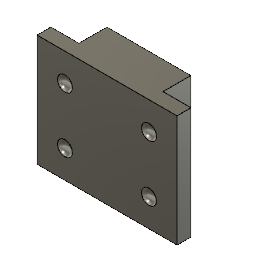
Open-JIP Plant Back Panel v1 (Autodesk Fusion 360 design; units mm, degrees)
Autodesk Fusion 360 part; units mm, degrees
sketch "Sketch1" plane through (0, 0, 0) normal (0, 1, 0) x (1, 0, 0)
  line L0 (0, 0) -> (100, 0)
  line L1 (100, 0) -> (100, 40)
  line L2 (100, 40) -> (0, 40)
  line L3 (0, 40) -> (0, 0)
  dimension "d1" = 100
  dimension "d2" = 40
  constraint horizontal L0
  constraint vertical L1
  constraint horizontal L2
  constraint vertical L3
  constraint coincident L0.start L3.end
  measures "d1" distance of L1.end L2.end
  measures "d2" distance of L0.end L1.end
extrude "Extrude1" add sketch "Sketch1" along normal blind 5 makes body 1
sketch "Sketch2" plane through (0, 5, 0) normal (0, 1, 0) x (-1, 0, 0)
  line L0 (0, -40) -> (0, 0)
  line L1 (0, 0) -> (-100, 0)
  line L2 (-100, 0) -> (-100, -40)
  line L3 (-100, -40) -> (0, -40)
  line L4 (0, -40) -> (-10, -40)
  line L5 (-10, -40) -> (-10, 0)
  line L6 (-10, 0) -> (0, 0)
  line L7 (0, 0) -> (0, -40)
  dimension "d5" = 10
  constraint horizontal L4
  constraint vertical L5
  constraint horizontal L6
  constraint vertical L7
  constraint coincident L1 L5.end
  constraint coincident L0.start L3.end
  measures "d5" distance of L0.start L4.end
extrude "Extrude2" add sketch "Sketch2" along normal blind 3 contours L0 L1 L3 L4 L5 L6 L7 bodies 1
sketch "Sketch3" plane through (0, 8, 0) normal (0, 1, 0) x (-1, 0, 0)
  line L0 (0, 0) -> (-10, 0)
  line L1 (-10, 0) -> (-10, -40)
  line L2 (-10, -40) -> (0, -40)
  line L3 (0, -40) -> (0, 0)
  line L4 (0, -40) -> (-100, -40)
  line L5 (-100, -40) -> (-100, 0)
  line L6 (-100, 0) -> (0, 0)
  line L7 (0, 0) -> (0, -40)
  point P0 (-100, 0)
  constraint horizontal L4
  constraint vertical L5
  constraint horizontal L6
  constraint vertical L7
  constraint coincident P0 L5.end
  constraint coincident L2.end L3.start
extrude "Extrude3" add sketch "Sketch3" along normal blind 6 bodies 1
sketch "Sketch4" plane through (100, 0, 0) normal (1, 0, 0) x (0, 0, -1)
  line L0 (0, 8) -> (40, 8)
  line L1 (40, 8) -> (40, 14)
  line L2 (40, 14) -> (0, 14)
  line L3 (0, 14) -> (0, 8)
  line L4 (2, 13) -> (38, 13)
  line L5 (38, 13) -> (38, 9)
  line L6 (38, 9) -> (2, 9)
  line L7 (2, 9) -> (2, 13)
  dimension "d10" = 4
  dimension "d11" = 2
  dimension "d12" = 2
  dimension "d13" = 1
  constraint horizontal L4
  constraint vertical L5
  constraint horizontal L6
  constraint vertical L7
  measures "d10" distance of L4.start L6.end
  measures "d11" distance of L1 L5
  measures "d12" distance of L3 L7
  measures "d13" distance of L0 L6
extrude "Extrude4" cut sketch "Sketch4" against normal blind 90 contours L4 L5 L6 L7 bodies 1
sketch "Sketch5" plane through (0, 14, 0) normal (0, 1, 0) x (-1, 0, 0)
  line L0 (0, 0) -> (-100, 0)
  line L1 (-100, 0) -> (-100, -40)
  line L2 (-100, -40) -> (0, -40)
  line L3 (0, -40) -> (0, 0)
  circle A0 centre (-55, -20) radius 7.5
  dimension "d16" = 20
  dimension "d17" = 15
  dimension "d18" = 55
  measures "d16" distance of L2 A0.centre
  measures "d17" diameter of A0
  measures "d18" distance of L3 A0.centre
extrude "Extrude5" cut sketch "Sketch5" against normal blind 8 contours A0 bodies 1
sketch "Sketch6" plane through (0, 14, 0) normal (0, 1, 0) x (-1, 0, 0)
  circle A0 centre (-55, -20) radius 7.5
  line L0 (0, 0) -> (-100, 0)
  line L1 (-100, 0) -> (-100, -40)
  line L2 (-100, -40) -> (0, -40)
  line L3 (0, -40) -> (0, 0)
  circle A1 centre (-55, -20) radius 15
  dimension "d21" = 30
  constraint concentric A0 A1
  measures "d21" diameter of A1
extrude "Extrude6" cut sketch "Sketch6" against normal blind 2 contours A1 bodies 1
extrude "Extrude7" add 1 faces at (10, 11.6667, -14) along direction (1, 0, 0) blind 90 on bodies 1 bodies 1
sketch "Sketch7" plane through (0, 0, -40) normal (0, 0, -1) x (-1, 0, 0)
  line L0 (-100, 0) -> (0, 0)
  line L1 (0, 0) -> (0, 14)
  line L2 (0, 14) -> (-100, 14)
  line L3 (-100, 14) -> (-100, 8)
  line L4 (-100, 8) -> (-10, 8)
  line L5 (-10, 8) -> (-10, 5)
  line L6 (-10, 5) -> (-100, 5)
  line L7 (-100, 5) -> (-100, 0)
  line L8 (-80, 12.5) -> (-30, 12.5)
  line L9 (-30, 12.5) -> (-30, 9.5)
  line L10 (-30, 9.5) -> (-80, 9.5)
  line L11 (-80, 9.5) -> (-80, 12.5)
  dimension "d26" = 1.5
  dimension "d27" = 1.5
  dimension "d28" = 20
  dimension "d29" = 30
  constraint horizontal L8
  constraint vertical L9
  constraint horizontal L10
  constraint vertical L11
  measures "d26" distance of L4 L10
  measures "d27" distance of L2 L8
  measures "d28" distance of L3 L11
  measures "d29" distance of L1 L9
extrude "Extrude8" cut sketch "Sketch7" against normal blind 37 contours L8 L9 L10 L11 bodies 1
extrude "Extrude9" cut 1 faces at (55.8396, 13, -15.821) along direction (0, -1, 0) blind 1 on bodies 1 bodies 1
sketch "Sketch8" plane through (0, 9.5, 0) normal (0, 1, 0) x (-1, 0, 0)
  line L0 (-80, -40) -> (-30, -40)
  line L1 (-30, -40) -> (-30, -3)
  line L2 (-30, -3) -> (-80, -3)
  line L3 (-80, -3) -> (-80, -40)
  circle A0 centre (-55, -20) radius 7.5
extrude "Extrude10" cut sketch "Sketch8" against normal blind 2 contours A0 bodies 1
move_body "Move1" bodies 1 to x (1, 0, 0) y (0, 0, 1) z (0, -1, 0) at (0, 0, -40)
move_body "Move2" bodies 1 to x (1, 0, 0) y (0, 1, 0) z (0, 0, 1) at (0, 0, 25)
sketch "Sketch9" plane through (0, 0, -15) normal (0, 0, -1) x (-1, 0, 0)
  line L0 (0, 0) -> (0, 40)
  line L1 (0, 40) -> (-100, 40)
  line L2 (-100, 40) -> (-100, 0)
  line L3 (-100, 0) -> (0, 0)
  circle A0 centre (-70, 30) radius 2.5
  circle A1 centre (-40, 30) radius 2.5
  circle A2 centre (-40, 10) radius 2.5
  circle A3 centre (-70, 10) radius 2.5
  dimension "d36" = 5
  dimension "d37" = 5
  dimension "d38" = 5
  dimension "d39" = 5
  dimension "d40" = 20
  dimension "d41" = 20
  dimension "d42" = 30
  dimension "d43" = 30
  dimension "d44" = 10
  dimension "d45" = 30
  measures "d36" diameter of A3
  measures "d37" diameter of A0
  measures "d38" diameter of A1
  measures "d39" diameter of A2
  measures "d40" distance of A1.centre A2.centre
  measures "d41" distance of A0.centre A3.centre
  measures "d42" distance of A0.centre A1.centre
  measures "d43" distance of A2.centre A3.centre
  measures "d44" distance of L3 A3.centre
  measures "d45" distance of L2 A3.centre
extrude "Extrude11" add sketch "Sketch9" along normal blind 2 contours A0 | A1 | A2 | A3 bodies 1
sketch "Sketch1 (2)" plane through (0, 0, 0) normal (0, 1, 0) x (1, 0, 0) in component "Attachment for IRWIN QuickGrip v0 v1"
  line L0 (0, 0) -> (40, 0)
  line L1 (40, 0) -> (40, 30)
  line L2 (40, 30) -> (0, 30)
  line L3 (0, 30) -> (0, 0)
  constraint horizontal L0
  constraint vertical L1
  constraint horizontal L2
  constraint vertical L3
  constraint coincident L0.start L3.end
extrude "Extrude1'" add sketch "Sketch1 (2)" along normal blind 10 separate body makes body 2 in component "Attachment for IRWIN QuickGrip v0 v1"
sketch "Sketch2 (2)" plane through (40, 0, 0) normal (1, 0, 0) x (0, 0, -1) in component "Attachment for IRWIN QuickGrip v0 v1"
  line L0 (0, 0) -> (30, 0)
  line L1 (30, 0) -> (30, 10)
  line L2 (30, 10) -> (0, 10)
  line L3 (0, 10) -> (0, 0)
  line L4 (7.3, 10) -> (22.7, 10)
  line L5 (22.7, 10) -> (22.7, 5.5)
  line L6 (22.7, 5.5) -> (7.3, 5.5)
  line L7 (7.3, 5.5) -> (7.3, 10)
  dimension "d3_1" = 15.4
  dimension "d4_1" = 4.5
  dimension "d5_1" = 7.3
  constraint horizontal L4
  constraint vertical L5
  constraint horizontal L6
  constraint vertical L7
  constraint collinear L2 L4
  measures "d3_1" distance of L5.end L6.end
  measures "d4_1" distance of L4.end L5.end
  measures "d5_1" distance of L3 L7
extrude "Extrude2'" cut sketch "Sketch2 (2)" against normal blind 35 contours L2 L4 L5 L6 L7 bodies 2 in component "Attachment for IRWIN QuickGrip v0 v1"
sketch "Sketch3 (2)" plane through (40, 0, 0) normal (1, 0, 0) x (0, 0, -1) in component "Attachment for IRWIN QuickGrip v0 v1"
  line L0 (7.3, 5.5) -> (7.3, 10)
  line L1 (7.3, 10) -> (0, 10)
  line L2 (0, 10) -> (0, 0)
  line L3 (0, 0) -> (30, 0)
  line L4 (30, 0) -> (30, 10)
  line L5 (30, 10) -> (22.7, 10)
  line L6 (22.7, 10) -> (22.7, 5.5)
  line L7 (22.7, 5.5) -> (7.3, 5.5)
  line L8 (4.5, 5.5) -> (25.5, 5.5)
  line L9 (25.5, 5.5) -> (25.5, 1.2)
  line L10 (25.5, 1.2) -> (4.5, 1.2)
  line L11 (4.5, 1.2) -> (4.5, 5.5)
  dimension "d8_1" = 21
  dimension "d9_1" = 4.5
  dimension "d10_1" = 4.3
  constraint horizontal L8
  constraint vertical L9
  constraint horizontal L10
  constraint vertical L11
  constraint collinear L7 L8
  measures "d8_1" distance of L9 L11
  measures "d9_1" distance of L2 L11
  measures "d10_1" distance of L8.end L9.end
extrude "Extrude3'" cut sketch "Sketch3 (2)" against normal blind 38 contours L7 L8 L9 L10 L11 bodies 2 in component "Attachment for IRWIN QuickGrip v0 v1"
sketch "Sketch10" plane through (0, 0, -76.0627) normal (0, 0, 1) x (1, 0, 0)
  line L0 (68.8222, 42.7595) -> (38.8222, 42.7595)
  line L1 (38.8222, 42.7595) -> (38.8222, 2.7595)
  line L2 (38.8222, 2.7595) -> (68.8222, 2.7595)
  line L3 (68.8222, 2.7595) -> (68.8222, 42.7595)
  line L4 (28.8222, 42.7595) -> (78.8222, 42.7595)
  line L5 (78.8222, 42.7595) -> (78.8222, 2.7595)
  line L6 (78.8222, 2.7595) -> (28.8222, 2.7595)
  line L7 (28.8222, 2.7595) -> (28.8222, 42.7595)
  dimension "d48" = 40
  dimension "d49" = 10
  dimension "d50" = 10
  constraint horizontal L4
  constraint vertical L5
  constraint horizontal L6
  constraint vertical L7
  measures "d48" distance of L4.end L5.end
  measures "d49" distance of L3 L5
  measures "d50" distance of L1 L7
extrude "Extrude4'" add sketch "Sketch10" along normal blind 5 sketch seen with x (0, 0, 1) y (-1, 0, 0) z (0, -1, 0) at (42.7595, -76.0627, -68.8222) bodies 2 in component "Attachment for IRWIN QuickGrip v0 v1"
sketch "Sketch11" plane through (0, 0, -71.0627) normal (0, 0, 1) x (1, 0, 0)
  line L0 (28.8222, 2.7595) -> (78.8222, 2.7595)
  line L1 (78.8222, 2.7595) -> (78.8222, 42.7595)
  line L2 (78.8222, 42.7595) -> (28.8222, 42.7595)
  line L3 (28.8222, 42.7595) -> (28.8222, 2.7595)
  circle A0 centre (38.8222, 32.7595) radius 2.65
  circle A1 centre (68.8222, 32.7595) radius 2.65
  circle A2 centre (68.8222, 12.7595) radius 2.65
  circle A3 centre (38.8222, 12.7595) radius 2.65
  dimension "d53" = 5.3
  dimension "d54" = 5.3
  dimension "d55" = 5.3
  dimension "d56" = 5.3
  dimension "d57" = 30
  dimension "d58" = 30
  dimension "d59" = 10
  dimension "d60" = 10
  dimension "d61" = 20
  dimension "d62" = 20
  dimension "d63" = 10
  dimension "d64" = 10
  measures "d53" diameter of A3
  measures "d54" diameter of A0
  measures "d55" diameter of A1
  measures "d56" diameter of A2
  measures "d57" horizontal distance of A0.centre A1.centre
  measures "d58" distance of A2.centre A3.centre
  measures "d59" distance of L3 A3.centre
  measures "d60" distance of L3 A0.centre
  measures "d61" distance of A1.centre A2.centre
  measures "d62" distance of A0.centre A3.centre
  measures "d63" distance of L2 A0.centre
  measures "d64" distance of L2 A1.centre
extrude "Extrude5'" cut sketch "Sketch11" against normal blind 2 contours A0 | A1 | A2 | A3 sketch seen with x (0, 0, 1) y (-1, 0, 0) z (0, -1, 0) at (42.7595, -76.0627, -68.8222) bodies 2 in component "Attachment for IRWIN QuickGrip v0 v1"
fillet "Fillet1" radius 2.5 4 edges at (72.3308, 29.096, -17) (72.3308, 9.096, -17) (42.3308, 9.096, -17) (42.3308, 29.096, -17) on bodies 1
fillet "Fillet1'" radius 2.6 4 edges at (9.0417, -3, -2.4707) (29.0417, -3, -2.4707) (29.0417, -3, -32.4707) (9.0417, -3, -32.4707) on bodies 2 in component "Attachment for IRWIN QuickGrip v0 v1"
sketch "Sketch12" plane through (0, 0, -1) normal (0, 0, 1) x (1, 0, 0)
  circle A0 centre (55, 20) radius 15
  line L0 (0, 0) -> (100, 0)
  line L1 (100, 0) -> (100, 40)
  line L2 (100, 40) -> (0, 40)
  line L3 (0, 40) -> (0, 0)
  line L4 (35, 35) -> (75, 35)
  line L5 (75, 35) -> (75, 5)
  line L6 (75, 5) -> (35, 5)
  line L7 (35, 5) -> (35, 35)
  constraint horizontal L4
  constraint vertical L5
  constraint horizontal L6
  constraint vertical L7
extrude "Extrude12" cut sketch "Sketch12" against normal blind 6 contours A0 | A0 L4 L5 L6 | A0 L4 L6 L7 bodies 1
sketch "Sketch13" plane through (0, 0, -1) normal (0, 0, 1) x (1, 0, 0)
  line L0 (35, 35) -> (75, 35)
  line L1 (75, 35) -> (75, 5)
  line L2 (75, 5) -> (35, 5)
  line L3 (35, 5) -> (35, 35)
  line L4 (0, 0) -> (100, 0)
  line L5 (100, 0) -> (100, 40)
  line L6 (100, 40) -> (0, 40)
  line L7 (0, 40) -> (0, 0)
  line L8 (100, 40) -> (92.558, 40)
  line L9 (92.558, 40) -> (92.558, 0)
  line L10 (92.558, 0) -> (100, 0)
  line L11 (100, 0) -> (100, 40)
  line L12 (20.442, 40) -> (12.942, 40)
  line L13 (12.942, 40) -> (12.942, 0)
  line L14 (12.942, 0) -> (20.442, 0)
  line L15 (20.442, 0) -> (20.442, 40)
  dimension "d83" = 87.058
  dimension "d84" = 7.442
  dimension "d85" = 7.5
  constraint horizontal L8
  constraint vertical L9
  constraint horizontal L10
  constraint vertical L11
  constraint coincident L4 L9.end
  constraint coincident L5.end L6.start
  constraint horizontal L12
  constraint vertical L13
  constraint horizontal L14
  constraint vertical L15
  constraint coincident L4 L13.end
  constraint coincident L6 L12.start
  measures "d83" distance of L11 L13
  measures "d84" distance of L9 L11
  measures "d85" distance of L13 L15
extrude "Extrude13" add sketch "Sketch13" along normal blind 12 contours L4 L6 L12 L13 L14 L15 | L4 L5 L6 L8 L9 L10 L11 bodies 1
fillet "Fillet2" radius 12 2 edges at (20.442, 20, -1) (92.558, 20, -1) on bodies 1
fillet "Fillet3" radius 14 1 edges at (12.942, 20, -1) on bodies 1
sketch "Sketch14" plane through (-1.1778, 2.7595, -71.0627) normal (0, 0, 1) x (1, 0, 0)
  circle A0 centre (70, 10) radius 2.65
  circle A1 centre (40, 10) radius 2.65
  circle A2 centre (70, 30) radius 2.65
  circle A3 centre (40, 30) radius 2.65
  line L0 (30, 0) -> (80, 0)
  line L1 (80, 0) -> (80, 40)
  line L2 (80, 40) -> (30, 40)
  line L3 (30, 40) -> (30, 0)
  line L4 (27, 40) -> (83, 40)
  line L5 (83, 40) -> (83, 0)
  line L6 (83, 0) -> (27, 0)
  line L7 (27, 0) -> (27, 40)
  dimension "d90" = 3
  dimension "d91" = 3
  dimension "d92" = 3
  dimension "d93" = 40
  constraint horizontal L4
  constraint vertical L5
  constraint horizontal L6
  constraint vertical L7
  measures "d90" distance of L1 L5
  measures "d91" distance of L0.start L6.end
  measures "d92" distance of L3 L7
  measures "d93" distance of L4 L6
sketch "Sketch15" plane through (0, 0, -65) normal (0, 0, -1) x (-1, 0, 0)
  line L0 (-83, 0) -> (-27, 0)
  line L1 (-27, 0) -> (-27, 40)
  line L2 (-27, 40) -> (-83, 40)
  line L3 (-83, 40) -> (-83, 0)
  line L4 (-83, 40) -> (-80.1, 40)
  line L5 (-80.1, 40) -> (-80.1, 0)
  line L6 (-80.1, 0) -> (-83, 0)
  line L7 (-83, 0) -> (-83, 40)
  line L8 (-27, 40) -> (-29.9, 40)
  line L9 (-29.9, 40) -> (-29.9, 0)
  line L10 (-29.9, 0) -> (-27, 0)
  line L11 (-27, 0) -> (-27, 40)
  dimension "d96" = 2.9
  dimension "d97" = 2.9
  constraint horizontal L4
  constraint vertical L5
  constraint horizontal L6
  constraint vertical L7
  constraint coincident L0 L5.end
  constraint coincident L2.end L3.start
  constraint horizontal L8
  constraint vertical L9
  constraint horizontal L10
  constraint vertical L11
  constraint coincident L0 L9.end
  constraint coincident L1.end L2.start
  measures "d96" distance of L5 L7
  measures "d97" distance of L9 L11
sketch "Sketch16" plane through (0, 0, -57) normal (0, 0, 1) x (1, 0, 0)
  line L0 (27, 0) -> (83, 0)
  line L1 (83, 0) -> (83, 40)
  line L2 (83, 40) -> (27, 40)
  line L3 (27, 40) -> (27, 0)
  circle A0 centre (55, 20) radius 4
  dimension "d100" = 8
  dimension "d101" = 20
  dimension "d102" = 28
  measures "d100" diameter of A0
  measures "d101" distance of L2 A0.centre
  measures "d102" distance of L3 A0.centre
component "Attachment for IRWIN QuickGrip v0 v1" placed x (0, -1, 0) y (0, 0, -1) z (1, 0, 0) at (68.8222, 42.7595, -76.0627)
hidden bodies 1
